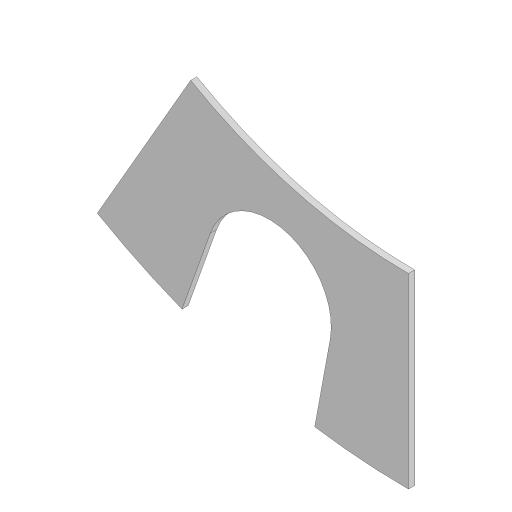
# Autodesk Inventor part: 円盤1
Saved by Autodesk Inventor 2023 (Build 270158000, 158)
## iProperties
Created: 2022-09-02
Part Number: 円盤1
Material: 一般
Document SubType Name: Modeling
Designer: monst
Density: 1 g/cm^3
Appearance: 既定
Author: monst
Autodesk Inventor part; units mm, degrees
ref_plane "YZ Plane" through (0, 0, 0) normal (1, 0, 0) x (0, 1, 0)
ref_plane "XZ Plane" through (0, 0, 0) normal (0, 1, 0) x (-1, 0, 0)
ref_plane "XY Plane" through (0, 0, 0) normal (0, 0, 1) x (1, 0, 0)
sketch "スケッチ1" plane through (0, 0, 0) normal (0, 0, 1) x (1, 0, 0)
  circle A0 centre (0, 0) radius 100
  circle A1 centre (0, 0) radius 70
  line L0 (0, 100) -> (50, 86.6025)
  line L1 (50, 86.6025) -> (86.6025, 50)
  line L2 (86.6025, 50) -> (100, 0)
  line L3 (100, 0) -> (86.6025, -50)
  line L4 (86.6025, -50) -> (50, -86.6025)
  line L5 (50, -86.6025) -> (0, -100)
  line L6 (0, -100) -> (-50, -86.6025)
  line L7 (-50, -86.6025) -> (-86.6025, -50)
  line L8 (-86.6025, -50) -> (-100, 0)
  line L9 (-100, 0) -> (-86.6025, 50)
  line L10 (-86.6025, 50) -> (-50, 86.6025)
  line L11 (-50, 86.6025) -> (0, 100)
  line L12 (0, 0) -> (-50, -86.6025)
  line L13 (0, -100) -> (0, 0)
  line L14 (-25, -93.3013) -> (0, 0)
  line L15 (-25, -93.3013) -> (-22.4118, -83.642)
  circle A2 centre (-22.4118, -83.642) radius 10
  line L16 (-22.4118, -83.642) -> (-32.0711, -81.0538)
  line L17 (-22.4118, -83.642) -> (-12.7526, -86.2302)
  line L18 (-22.4118, -83.642) -> (-28.8823, -107.7902)
  line L19 (-28.8823, -107.7902) -> (-40.4734, -104.6843)
  line L20 (-40.4734, -104.6843) -> (-31.838, -80.3034)
  line L21 (-28.8823, -107.7902) -> (-17.2912, -110.896)
  line L22 (-17.2912, -110.896) -> (-12.5792, -85.4638)
  point P0 (0, -100)
  point P1 (0, -70)
  point P2 (-35, -60.6218)
  point P3 (-25, -93.3013)
  point P4 (-36.3864, -93.1452)
  point P5 (-15.061, -98.8593)
  dimension "d0" = 200
  dimension "d1" = 140
  dimension "d2" = 10
  dimension "d3" = 20
  dimension "d4" = 90
  dimension "d5" = 90
  dimension "d8" = 25
  dimension "d9" = 12
  dimension "d10" = 12
  constraints: 46 end point, 4 coincident, 4 point on circle, 2 centre point, 2 point on line, 2 tangent, 1 midpoint, 1 perpendicular, 1 vertical, 28 other
  measures "d1" diameter of A1
  measures "d2" distance of L14.start L15.end
  measures "d3" diameter of A2
  measures "d4" angle of L14 L17
  measures "d5" angle of L14 L16
  measures "d8" distance of L15.end L18.end
  measures "d9" distance of L18.end L19.end
  measures "d10" distance of L18.end L21.end
extrude "押し出し2" add sketch "スケッチ1" along normal blind 1 contours A0 L22 L6 | L6 L22 A2 L14 A1 L13 | L14 A2 L20 L6 L12 A1 | A0 L6 L20
